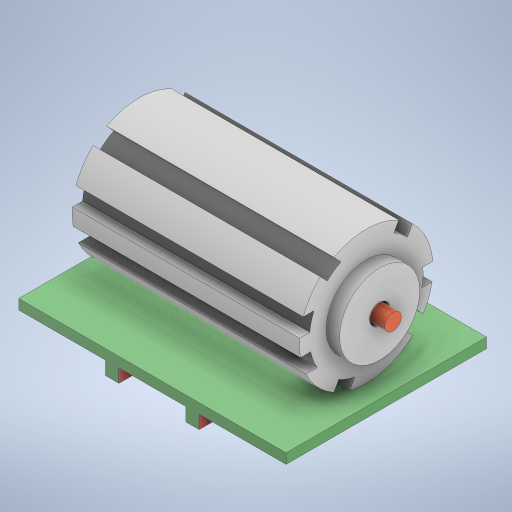
# Autodesk Inventor part: motor
Saved by Autodesk Inventor 2023 (Build 270158000, 158)
## iProperties
Created: 2022-04-04
Part Number: motor
Material: Genérico
Document SubType Name: Modeling
Designer: isaac
Density: 1 g/cm^3
Appearance: Valor por defecto
Author: isaac
Autodesk Inventor part; units mm, degrees
ref_plane "YZ Plane" through (0, 0, 0) normal (1, 0, 0) x (0, 1, 0)
ref_plane "XZ Plane" through (0, 0, 0) normal (0, 1, 0) x (-1, 0, 0)
ref_plane "XY Plane" through (0, 0, 0) normal (0, 0, 1) x (1, 0, 0)
sketch "Boceto1" plane through (0, 0, 0) normal (0, 1, 0) x (-1, 0, 0)
  line L0 (200, 150) -> (-200, 150)
  line L1 (-200, 150) -> (-200, -150)
  line L2 (-200, -150) -> (200, -150)
  line L3 (200, -150) -> (200, 150)
  point P0 (0, 0)
  point P1 (200, 0)
  point P2 (0, -150)
  dimension "d0" = 300
  dimension "d1" = 400
  constraints: 8 end point, 2 midpoint, 2 parallel, 1 horizontal, 1 horizontal alignment, 1 perpendicular, 1 vertical alignment
  measures "d0" distance between parallel lines of L2 L0
  measures "d1" distance between parallel lines of L1 L3
extrude "Extrusión1" add sketch "Boceto1" along normal blind 15
sketch "Boceto2" plane through (0, 0, 0) normal (1, 0, 0) x (0, 1, 0)
  line L0 (0, -150) -> (0, 150) construction
  line L1 (0, 150) -> (15, 150) construction
  line L2 (15, -150) -> (15, 150) construction
  line L3 (0, -150) -> (15, -150) construction
  circle A0 centre (115, 0) radius 85
  line L4 (187.5593, 68.8124) -> (176.6978, 58.467)
  line L5 (202.4618, 48.4812) -> (191.1695, 37.7255)
  line L6 (73.6141, -74.2442) -> (62.3217, -85)
  line L7 (27.5235, 48.4548) -> (40.6428, 41.1826)
  line L8 (189.3279, -41.2355) -> (202.4471, -48.5077)
  line L9 (123.3693, 99.6492) -> (123.3693, 84.587)
  line L10 (148.3693, 94.2682) -> (148.3693, 78.176)
  line L11 (148.3693, -78.176) -> (148.3693, -94.2682)
  line L12 (173.9112, -61.2738) -> (187.5427, -68.8299)
  line L13 (123.3693, -84.587) -> (123.3693, -99.6492)
  line L14 (97.5795, 98.4709) -> (97.5795, 83.1957)
  line L15 (72.5795, 90.5566) -> (72.5795, 73.658)
  line L16 (72.5795, -73.658) -> (72.5795, -75.2297)
  line L17 (18.1873, 25.046) -> (31.8189, 17.4899)
  line L18 (53.6011, -58.7807) -> (42.7395, -69.1261)
  line L19 (97.5795, -83.1957) -> (97.5795, -98.4709)
  arc A1 (187.5593, 68.8124) -> (148.3693, 94.2682) centre (115, 0) ccw
  arc A2 (123.3693, 99.6492) -> (97.5795, 98.4709) centre (115, 0) ccw
  arc A3 (72.5795, 90.5566) -> (27.5235, 48.4548) centre (115, 0) ccw
  arc A4 (18.1873, 25.046) -> (42.7395, -69.1261) centre (115, 0) ccw
  arc A5 (62.3217, -85) -> (97.5795, -98.4709) centre (115, 0) ccw
  arc A6 (123.3693, -99.6492) -> (187.5427, -68.8299) centre (115, 0) ccw
  arc A7 (202.4471, -48.5077) -> (202.4618, 48.4812) centre (115, 0) ccw
  point P0 (0, 0)
  point P1 (0, 0)
  dimension "d5" = 170
  constraints: 32 end point, 15 point on circle, 10 parallel, 7 centre point, 4 vertical, 1 coincident, 1 horizontal alignment, 1 midpoint, 1 point on line, 1 tangent, 18 other
extrude "Extrusión2" add sketch "Boceto2" along normal mid plane 340 contours A0 | A0 L5 A7 L8 | A0 L10 A1 L4 | L12 A6 L11 A0 | L11 A6 L13 A0 | A0 L14 A2 L9 | L19 A5 L6 A0 | A0 L7 A3 L15 | A0 L18 A4 L17
sketch "Boceto3" plane through (170, 0, 0) normal (1, 0, 0) x (0, 0, -1)
  line L0 (-48.4812, 202.4618) -> (-37.7255, 191.1695) construction
  arc A0 (-37.7255, 191.1695) -> (-58.467, 176.6978) centre (0, 115) ccw construction
  line L1 (-58.467, 176.6978) -> (-68.8124, 187.5593) construction
  arc A1 (-68.8124, 187.5593) -> (-94.2682, 148.3693) centre (0, 115) ccw construction
  line L2 (-94.2682, 148.3693) -> (-78.176, 148.3693) construction
  arc A2 (-78.176, 148.3693) -> (-84.587, 123.3693) centre (0, 115) ccw construction
  line L3 (-84.587, 123.3693) -> (-99.6492, 123.3693) construction
  arc A3 (-99.6492, 123.3693) -> (-98.4709, 97.5795) centre (0, 115) ccw construction
  line L4 (-98.4709, 97.5795) -> (-83.1957, 97.5795) construction
  arc A4 (-83.1957, 97.5795) -> (-73.658, 72.5795) centre (0, 115) ccw construction
  line L5 (-73.658, 72.5795) -> (-90.5566, 72.5795) construction
  arc A5 (-90.5566, 72.5795) -> (-48.4548, 27.5235) centre (0, 115) ccw construction
  line L6 (-48.4548, 27.5235) -> (-41.1826, 40.6428) construction
  arc A6 (-41.1826, 40.6428) -> (-17.4899, 31.8189) centre (0, 115) ccw construction
  line L7 (-17.4899, 31.8189) -> (-25.046, 18.1873) construction
  arc A7 (-25.046, 18.1873) -> (0, 15) centre (0, 115) ccw construction
  arc A8 (0, 15) -> (69.1261, 42.7395) centre (0, 115) ccw construction
  line L8 (69.1261, 42.7395) -> (58.7807, 53.6011) construction
  arc A9 (58.7807, 53.6011) -> (74.2442, 73.6141) centre (0, 115) ccw construction
  line L9 (74.2442, 73.6141) -> (85, 62.3217) construction
  arc A10 (85, 62.3217) -> (98.4709, 97.5795) centre (0, 115) ccw construction
  line L10 (98.4709, 97.5795) -> (83.1957, 97.5795) construction
  arc A11 (83.1957, 97.5795) -> (84.587, 123.3693) centre (0, 115) ccw construction
  line L11 (84.587, 123.3693) -> (99.6492, 123.3693) construction
  arc A12 (99.6492, 123.3693) -> (68.8299, 187.5427) centre (0, 115) ccw construction
  line L12 (68.8299, 187.5427) -> (61.2738, 173.9112) construction
  arc A13 (61.2738, 173.9112) -> (41.2355, 189.3279) centre (0, 115) ccw construction
  line L13 (41.2355, 189.3279) -> (48.5077, 202.4471) construction
  arc A14 (48.5077, 202.4471) -> (-48.4812, 202.4618) centre (0, 115) ccw construction
  circle A15 centre (0, 115) radius 60
  line L14 (-150, 15) -> (150, 15) projected
  point P0 (0, 0)
  dimension "d14" = 120
  dimension "d15" = 100
  constraints: 1 centre point, 1 coincident, 1 midpoint
  measures "d14" diameter of A15
  measures "d15" distance of point (0, 15) A15.centre
extrude "Extrusión3" add sketch "Boceto3" along normal blind 20
sketch "Boceto4" plane through (190, 115, 0) normal (1, 0, 0) x (0, 0, -1)
  circle A0 centre (0, 0) radius 15
  circle A1 centre (0, 0) radius 60 construction
  point P0 (0, -115)
  dimension "d18" = 30
  constraints: 2 coincident, 1 centre point
  measures "d18" diameter of A0
extrude "Extrusión4" cut sketch "Boceto4" against normal through all
sketch "Boceto5" plane through (190, 115, 0) normal (1, 0, 0) x (0, 0, -1)
  circle A0 centre (0, 0) radius 15 construction
  circle A1 centre (0, 0) radius 60 construction
  circle A2 centre (0, 0) radius 12.5
  point P0 (0, -115)
  dimension "d21" = 25
  constraints: 1 centre point, 1 coincident
  measures "d21" diameter of A2
extrude "Extrusión5" add sketch "Boceto5" along normal blind 20 and the other way blind 370
sketch "Boceto7" plane through (0, 0, 0) normal (0, -1, 0) x (1, 0, 0)
  line L0 (200, 150) -> (200, -150) construction
  line L1 (-200, 150) -> (200, 150) construction
  line L2 (-200, -150) -> (-200, 150) construction
  line L3 (200, -150) -> (-200, -150) construction
  line L4 (-200, 150) -> (200, 150) construction
  line L5 (-50, 150) -> (50, 150) construction
  line L6 (50, 150) -> (50, -150) construction
  line L7 (50, -150) -> (-50, -150) construction
  line L8 (-50, -150) -> (-50, 150) construction
  line L9 (200, -150) -> (-200, -150) projected
  line L10 (-50, 150) -> (-70, 150)
  line L11 (-70, 150) -> (-70, -150)
  line L12 (-70, -150) -> (-50, -150)
  line L13 (-50, -150) -> (-50, 150)
  line L14 (50, -150) -> (70, -150)
  line L15 (70, -150) -> (70, 150)
  line L16 (70, 150) -> (50, 150)
  line L17 (50, 150) -> (50, -150)
  point P0 (0, 0)
  point P1 (0, -150)
  dimension "d30" = 100
  dimension "d31" = 0
  dimension "d32" = 20
  dimension "d33" = 20
  constraints: 24 end point, 6 parallel, 3 horizontal, 3 perpendicular, 3 point on line, 1 midpoint, 1 vertical alignment
  measures "d30" distance between parallel lines of L6 L8
  measures "d31" distance between parallel lines of L3 L7
  measures "d32" distance between parallel lines of L8 L11
  measures "d33" distance between parallel lines of L6 L15
extrude "Extrusión7" add sketch "Boceto7" along normal blind 20
